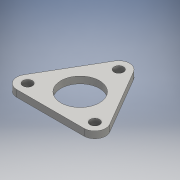
# Autodesk Inventor part: 240412_sketch2
Saved by Autodesk Inventor 2016 (Build 200138000, 138)
## iProperties
Created: 2024-04-12
Part Number: 240412_sketch2
Material: 일반
Document SubType Name: Modeling
Designer: pc
Density: 1 g/cm^3
Appearance: 기본값
Author: pc
Autodesk Inventor part; units mm, degrees
ref_plane "YZ Plane" through (0, 0, 0) normal (1, 0, 0) x (0, 1, 0)
ref_plane "XZ Plane" through (0, 0, 0) normal (0, 1, 0) x (-1, 0, 0)
ref_plane "XY Plane" through (0, 0, 0) normal (0, 0, 1) x (1, 0, 0)
sketch "스케치1" plane through (0, 0, 0) normal (0, 0, 1) x (1, 0, 0)
  circle A0 centre (0, 0) radius 28.5
  line L0 (0, 20.304) -> (0, -24.0188)
  line L1 (-22.2174, 0) -> (23.7675, 0)
  circle A1 centre (0, 57) radius 7
  circle A2 centre (-49.6488, -28) radius 7
  circle A3 centre (49.6488, -28) radius 7
  arc A4 (13.8158, 65.0699) -> (-13.8158, 65.0699) centre (0, 57) ccw
  arc A5 (-63.4646, -19.9301) -> (-49.6488, -44) centre (-49.6488, -28) ccw
  arc A6 (49.6488, -44) -> (63.4646, -19.9301) centre (49.6488, -28) ccw
  line L2 (-13.8158, 65.0699) -> (-63.4646, -19.9301)
  line L3 (13.8158, 65.0699) -> (63.4646, -19.9301)
  line L4 (-49.6488, -44) -> (49.6488, -44)
  arc A7 (-52.7065, -21.7031) -> (-45.8423, -33.8746) centre (0, 0) ccw
  dimension "d0" = 57
  dimension "d4" = 14
  dimension "d6" = 14
  dimension "d7" = 28
  dimension "d8" = 32
  dimension "d9" = 32
  dimension "d10" = 32
  constraints: 11 point on circle, 10 end point, 8 centre point, 5 coincident, 2 horizontal, 2 tangent, 1 point on line, 1 symmetric about line, 1 vertical
  measures "d0" diameter of A0
  measures "d4" diameter of A1
  measures "d6" diameter of A2
  measures "d7" vertical distance of A0.centre A2.centre
  measures "d8" diameter of A4
  measures "d9" diameter of A5
  measures "d10" diameter of A6
extrude "돌출1" add sketch "스케치1" along normal blind 10
